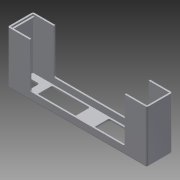
# Autodesk Inventor part: termination_hv_cover
Saved by Autodesk Inventor 2014 SP1 (Build 180222100, 222)
## iProperties
Created: 2016-10-04
Part Number: termination_hv_cover
Material: ABS Plastic
Document SubType Name: Modeling
Designer: tguillod
Density: 1.06 g/cm^3
Appearance: Smooth - White
Author: tguillod
Autodesk Inventor part; units mm, degrees
ref_plane "YZ Plane" through (0, 0, 0) normal (1, 0, 0) x (0, 1, 0)
ref_plane "XZ Plane" through (0, 0, 0) normal (0, 1, 0) x (-1, 0, 0)
ref_plane "XY Plane" through (0, 0, 0) normal (0, 0, 1) x (1, 0, 0)
sketch "Sketch1" plane through (0, 0, 0) normal (0, 0, 1) x (1, 0, 0)
  line L0 (0, 0) -> (29.75, 0)
  line L1 (29.75, 0) -> (29.75, 16)
  line L2 (29.75, 16) -> (0, 16)
  line L3 (0, 16) -> (0, 0)
  dimension "d0" = 16
  dimension "d1" = 29.75
  constraints: 8 end point, 2 parallel, 1 horizontal, 1 perpendicular
  measures "d0" distance of L0.end L1.end
  measures "d1" distance of L1.end L2.end
extrude "Extrusion1" add sketch "Sketch1" along normal blind 5
sketch "Sketch2" plane through (0, 0, 0) normal (0, 0, -1) x (-1, 0, 0)
  line L0 (0, 0) -> (-29.75, 0) projected
  line L1 (-29.75, 16) -> (-43.75, 16)
  line L2 (-43.75, 16) -> (-43.75, 0)
  line L3 (-43.75, 0) -> (-29.75, 0)
  line L4 (-29.75, 0) -> (-29.75, 16)
  dimension "d4" = 14
  constraints: 8 end point, 2 parallel, 1 collinear, 1 horizontal, 1 perpendicular
  measures "d4" distance of L1.start L1.end
extrude "Extrusion2" add sketch "Sketch2" against normal blind 33
sketch "Sketch4" plane through (0, 0, 33) normal (0, 0, 1) x (1, 0, 0)
  line L0 (43.75, 16) -> (29.75, 16) projected
  line L1 (29.75, 0) -> (43.75, 0) projected
  line L2 (43.75, 0) -> (43.75, 16) projected
  line L3 (42.75, 15) -> (0, 15)
  line L4 (0, 15) -> (0, 1)
  line L5 (0, 1) -> (42.75, 1)
  line L6 (42.75, 1) -> (42.75, 15)
  line L7 (0, 16) -> (0, 0) projected
  dimension "d14" = 1
  dimension "d15" = 1
  dimension "d16" = 1
  constraints: 8 end point, 2 parallel, 1 collinear, 1 horizontal, 1 perpendicular
  measures "d14" distance between parallel lines of L0 L3
  measures "d15" distance between parallel lines of L2 L6
  measures "d16" distance between parallel lines of L5 L1
extrude "Extrusion4" cut sketch "Sketch4" against normal blind 32
sketch "Sketch5" plane through (0, 0, 0) normal (0, 0, -1) x (-1, 0, 0)
  line L0 (0, 16) -> (0, 0) projected
  line L1 (-43.75, 16) -> (-43.75, 0) projected
  line L2 (-29.75, 14) -> (-6, 14)
  line L3 (-6, 14) -> (-6, 2)
  line L4 (-6, 2) -> (-29.75, 2)
  line L5 (-29.75, 2) -> (-29.75, 14)
  line L6 (-29.75, 14) -> (-6, 2) construction
  line L7 (-6, 14) -> (-29.75, 2) construction
  line L8 (-43.75, 8) -> (0, 8) construction
  point P0 (-17.875, 8)
  point P1 (-17.875, 8)
  dimension "d19" = 23.75
  dimension "d20" = 12
  dimension "d21" = 14
  constraints: 14 end point, 5 midpoint, 2 parallel, 1 horizontal, 1 perpendicular, 1 point on line
  measures "d19" distance of L2.start L2.end
  measures "d20" distance of L2.end L3.end
  measures "d21" distance between parallel lines of L1 L5
extrude "Extrusion5" cut sketch "Sketch5" against normal blind 15
sketch "Sketch10" plane through (42.75, 1, 33) normal (-1, 0, 0) x (0, 0, 1)
  line L0 (0, 14) -> (0, 0) projected
  line L1 (0, 14) -> (-32, 14) projected
  line L2 (0, 0) -> (-32, 0) projected
  line L3 (-1, 14) -> (-2, 14)
  line L4 (-2, 14) -> (-2, 0)
  line L5 (-2, 0) -> (-1, 0)
  line L6 (-1, 0) -> (-1, 14)
  point P0 (-33, -1)
  dimension "d63" = 1
  dimension "d64" = 1
  constraints: 8 end point, 2 parallel, 2 point on line, 1 horizontal, 1 perpendicular
  measures "d63" distance of L3.start L3.end
  measures "d64" distance between parallel lines of L0 L6
extrude "Extrusion10" add sketch "Sketch10" along normal blind 1 contours L6 L2 L4 L1
fillet "Fillet17" radius 1 2 edges at (29.75, 15.5, 5) (29.75, 0.5, 5)
fillet "Fillet18" radius 1 4 edges at (29.75, 2, 0.5) (29.75, 14, 0.5) (6, 14, 0.5) (6, 2, 0.5)
fillet "Fillet19" radius 1 5 edges at (43.75, 0, 16.5) (43.75, 16, 16.5) (21.875, 16, 0) (43.75, 8, 0) (21.875, 0, 0)
sketch "Sketch11" plane through (0, 0, 0) normal (0, 0, -1) x (-1, 0, 0)
  line L0 (-42.75, 1) -> (-42.75, 15) projected
  line L1 (0, 15) -> (0, 1) projected
  line L2 (-42.75, 8) -> (0, 8) construction
  line L3 (-39.75, 11) -> (-35.75, 11)
  line L4 (-34.75, 10) -> (-34.75, 6)
  line L5 (-35.75, 5) -> (-39.75, 5)
  line L6 (-40.75, 6) -> (-40.75, 10)
  line L7 (-40.75, 11) -> (-34.75, 5) construction
  line L8 (-34.75, 11) -> (-40.75, 5) construction
  arc A0 (-39.75, 11) -> (-40.75, 10) centre (-39.75, 10) ccw
  arc A1 (-34.75, 10) -> (-35.75, 11) centre (-35.75, 10) ccw
  arc A2 (-35.75, 5) -> (-34.75, 6) centre (-35.75, 6) ccw
  arc A3 (-40.75, 6) -> (-39.75, 5) centre (-39.75, 6) ccw
  point P0 (0, 0)
  point P1 (-37.75, 8)
  dimension "d71" = 6
  dimension "d72" = 6
  dimension "d73" = 2
  dimension "d74" = 1
  constraints: 14 end point, 9 point on line, 8 point on circle, 8 tangent, 4 centre point, 4 midpoint, 3 equal radius, 2 parallel, 1 horizontal, 1 perpendicular
  measures "d71" distance of L7.start L8.start
  measures "d72" distance of L8.start L7.end
  measures "d73" distance between parallel lines of L0 L6
  measures "d74" radius of A0
extrude "Extrusion11" cut sketch "Sketch11" against normal blind 10
mirror "Mirror1" about plane through (0, 16, 0) normal (-1, 0, 0)
body "Solid1"
